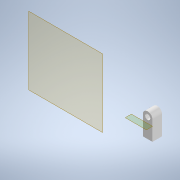
# Autodesk Inventor part: Falange_proxima
Saved by Autodesk Inventor 2020 (Build 240168000, 168)
## iProperties
Created: 2021-08-17
Part Number: Falange_proxima
Material: Generic
Document SubType Name: Modeling
Designer: chalo
Density: 1 g/cm^3
Appearance: Default
Author: chalo
Autodesk Inventor part; units mm, degrees
ref_plane "YZ Plane" through (0, 0, 0) normal (1, 0, 0) x (0, 1, 0)
ref_plane "XZ Plane" through (0, 0, 0) normal (0, 1, 0) x (-1, 0, 0)
ref_plane "XY Plane" through (0, 0, 0) normal (0, 0, 1) x (1, 0, 0)
ref_plane "Work Plane1" through (0, 0, 0) normal (0, 0, 1) x (-1, 0, 0)
sketch "Sketch1" plane through (0, 0, 0) normal (0, 0, 1) x (-1, 0, 0)
  circle A0 centre (-62.35, -16.0354) radius 1.6 projected
  circle A1 centre (-62.35, -16.0354) radius 3
  point P0 (0, 0)
  dimension "d0" = 6
  constraints: 1 centre point, 1 coincident
  measures "d0" diameter of A1
extrude "Extrusion1" add sketch "Sketch1" along normal mid plane 6
ref_plane "Work Plane2" through (57.35, 11.5354, 7.25) normal (0, -1, 0) x (1, 0, 0)
sketch "Sketch2" plane through (57.35, 11.5354, 7.25) normal (0, -1, 0) x (1, 0, 0)
  line L0 (2, -10.25) -> (8, -10.25) projected
  line L1 (8, -4.25) -> (2, -4.25) projected
  line L2 (2, -4.25) -> (8, -4.25)
  line L3 (8, -4.25) -> (8, -10.25)
  line L4 (8, -10.25) -> (2, -10.25)
  line L5 (2, -10.25) -> (2, -4.25)
  point P0 (-57.35, -7.25)
  constraints: 8 end point, 2 parallel, 1 horizontal, 1 perpendicular
extrude "Extrusion2" add sketch "Sketch2" along normal up to surface round surface about axis through (62.35, 16.0354, 0) along (0, 0, 1) radius 3 far side no
sketch "Sketch3" plane through (57.35, 11.5354, 7.25) normal (0, -1, 0) x (1, 0, 0)
  line L0 (8, -4.25) -> (2, -4.25) projected
  line L1 (2, -4.25) -> (2, -10.25) projected
  line L2 (2, -10.25) -> (8, -10.25) projected
  line L3 (8, -10.25) -> (8, -4.25) projected
  point P0 (-57.35, -7.25)
extrude "Extrusion3" add sketch "Sketch3" along normal blind 9
sketch "Sketch4" plane through (65.35, 16.0354, 3) normal (1, 0, 0) x (0, 0, -1)
  circle A0 centre (3, -4.76) radius 11.1046 construction
  circle A1 centre (3, -4.76) radius 10
  circle A2 centre (3, -4.76) radius 7
  line L0 (-4.75, -1.6) -> (-0.75, -1.6) construction
  line L1 (6.75, -1.6) -> (10.75, -1.6) construction
  line L2 (-4.75, -3) -> (-0.75, -3) construction
  line L3 (10.75, -3) -> (6.75, -3) construction
  line L4 (-3.7751, -3) -> (-6.8439, -3)
  line L5 (9.7751, -3) -> (12.8439, -3)
  point P0 (3, -16.0354)
  dimension "d7" = 20
  dimension "d8" = 14
  constraints: 8 end point, 4 point on circle, 4 point on line, 2 centre point, 2 coincident, 2 horizontal, 4 other
  measures "d7" diameter of A1
  measures "d8" diameter of A2
extrude "Extrusion4" add sketch "Sketch4" along normal blind 2.5 and the other way blind 7.5 contours A1 L4 A2 L5 picked at (11.9068, -5.5427)
sketch "Sketch5" plane through (67.85, 16.0354, 3) normal (1, 0, 0) x (0, 0, -1)
  arc A0 (-6.8439, -3) -> (12.8439, -3) centre (3, -4.76) ccw projected
  line L0 (12.8439, -3) -> (9.7751, -3) projected
  arc A1 (-3.7751, -3) -> (9.7751, -3) centre (3, -4.76) ccw projected
  line L1 (-3.7751, -3) -> (-6.8439, -3) projected
  point P0 (3, -16.0354)
extrude "Extrusion5" add sketch "Sketch5" along normal blind 12
body "Solid1"
